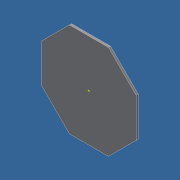
# Autodesk Inventor part: Oktagon_Deckel
Saved by Autodesk Inventor 2018.2 (Build 222227000, 227)
## iProperties
Created: 2018-10-01
Part Number: Oktagon_Deckel
Material: geeigneten Werkstoff auswählen !
Document SubType Name: Modeling
Designer: N.Grubert
Density: 0.001 g/cm^3
Appearance: Vorgabe
Fläche: 0 cm²
Gewicht: 0 g
Dateiname: P:\INVENTOR\Inventor 2018\Templates\ILT\Norm.ipt
Bez_eng: bolt
Bez_french: boulon
Author: N.Grubert
Autodesk Inventor part; units mm, degrees
ref_plane "YZ Plane" through (0, 0, 0) normal (1, 0, 0) x (0, 1, 0)
ref_plane "XZ Plane" through (0, 0, 0) normal (0, 1, 0) x (-1, 0, 0)
ref_plane "XY Plane" through (0, 0, 0) normal (0, 0, 1) x (1, 0, 0)
sketch "Skizze4" plane through (0, 0, 0) normal (0, 1, 0) x (-1, 0, 0)
  line L0 (22.7817, 55) -> (55, 22.7817)
  line L1 (55, 22.7817) -> (55, -22.7817)
  line L2 (55, -22.7817) -> (22.7817, -55)
  line L3 (22.7817, -55) -> (-22.7817, -55)
  line L4 (-22.7817, -55) -> (-55, -22.7817)
  line L5 (-55, -22.7817) -> (-55, 22.7817)
  line L6 (-55, 22.7817) -> (-22.7817, 55)
  line L7 (-22.7817, 55) -> (22.7817, 55)
  line L8 (0, -77) -> (0, 77) construction
  line L9 (77, 0) -> (-77, 0) construction
  point P0 (0, 0)
  point P1 (0, 0)
  dimension "d4" = 110
  constraints: 16 end point, 1 coincident, 18 other
  measures "d4" distance between parallel lines of L3 L7
extrude "Extrusion2" add sketch "Skizze4" along normal blind 2.5
